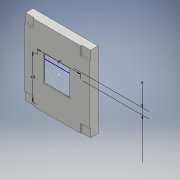
# Autodesk Inventor part: base
Saved by Autodesk Inventor 2018 (Build 220112000, 112)
## iProperties
Created: 2019-05-14
Part Number: base
Material: Generic
Document SubType Name: Modeling
Designer: jstklein
Density: 1 g/cm^3
Appearance: Default
Author: jstklein
Autodesk Inventor part; units mm, degrees
ref_plane "YZ Plane" through (0, 0, 0) normal (1, 0, 0) x (0, 1, 0)
ref_plane "XZ Plane" through (0, 0, 0) normal (0, 1, 0) x (-1, 0, 0)
ref_plane "XY Plane" through (0, 0, 0) normal (0, 0, 1) x (1, 0, 0)
sketch "Sketch1" plane through (0, 0, 0) normal (0, 1, 0) x (-1, 0, 0)
  line L0 (-30, 35) -> (30, 35)
  line L1 (30, 35) -> (30, -35)
  line L2 (30, -35) -> (-30, -35)
  line L3 (-30, -35) -> (-30, 35)
  line L4 (-30, 35) -> (30, -35) construction
  line L5 (30, 35) -> (-30, -35) construction
  point P0 (0, 0)
  dimension "d0" = 60
  dimension "d1" = 70
  constraints: 12 end point, 2 midpoint, 2 parallel, 1 horizontal, 1 perpendicular
  measures "d0" distance of L0.start L0.end
  measures "d1" distance of L0.end L1.end
extrude "Extrusion1" add sketch "Sketch1" along normal blind 8
sketch "Sketch2" plane through (0, 8, 0) normal (0, 1, 0) x (1, 0, 0)
  line L0 (27, -32) -> (27, 32)
  line L1 (27, 32) -> (-27, 32)
  line L2 (-27, 32) -> (-27, -32)
  line L3 (-27, -32) -> (27, -32)
  line L4 (27, -32) -> (-27, 32) construction
  line L5 (27, 32) -> (-27, -32) construction
  point P0 (0, 0)
  dimension "d4" = 64
  dimension "d5" = 54
  constraints: 12 end point, 2 midpoint, 2 parallel, 1 perpendicular, 1 vertical
  measures "d4" distance of L0.start L0.end
  measures "d5" distance of L1.end L0.end
extrude "Extrusion2" cut sketch "Sketch2" against normal blind 6
sketch "Sketch3" plane through (0, 2, 0) normal (0, 1, 0) x (1, 0, 0)
  line L0 (-12, -12) -> (12, -12)
  line L1 (12, -12) -> (12, 12)
  line L2 (12, 12) -> (-12, 12)
  line L3 (-12, 12) -> (-12, -12)
  line L4 (-12, -12) -> (12, 12) construction
  line L5 (12, -12) -> (-12, 12) construction
  line L6 (-13, -13) -> (13, -13)
  line L7 (13, -13) -> (13, 13)
  line L8 (13, 13) -> (-13, 13)
  line L9 (-13, 13) -> (-13, -13)
  line L10 (-13, -13) -> (13, 13) construction
  line L11 (13, -13) -> (-13, 13) construction
  circle A0 centre (-13, -13) radius 1.5
  circle A1 centre (-13, 13) radius 1.5
  circle A2 centre (13, 13) radius 1.5
  circle A3 centre (13, -13) radius 1.5
  point P0 (0, 0)
  dimension "d8" = 24
  dimension "d9" = 24
  dimension "d10" = 26
  dimension "d11" = 26
  dimension "d23" = 3
  dimension "d24" = 3
  dimension "d25" = 3
  dimension "d26" = 3
  constraints: 24 end point, 4 centre point, 4 coincident, 4 midpoint, 4 parallel, 2 horizontal, 2 perpendicular
  measures "d8" distance of L2.end L1.end
  measures "d9" distance of L1.end L0.end
  measures "d10" distance of L8.end L7.end
  measures "d11" distance of L7.end L6.end
  measures "d23" diameter of A0
  measures "d24" diameter of A1
  measures "d25" diameter of A2
  measures "d26" diameter of A3
extrude "Extrusion3" cut sketch "Sketch3" against normal blind 1.5
sketch "Sketch4" plane through (0, 0.5, 0) normal (0, 1, 0) x (1, 0, 0)
  line L0 (-12, -12) -> (12, -12)
  line L1 (12, -12) -> (12, 12)
  line L2 (12, 12) -> (-12, 12)
  line L3 (-12, 12) -> (-12, -12)
  line L4 (-12, -12) -> (12, 12) construction
  line L5 (12, -12) -> (-12, 12) construction
  point P0 (0, 0)
  dimension "d18" = 24
  dimension "d19" = 24
  constraints: 12 end point, 2 midpoint, 2 parallel, 1 horizontal, 1 perpendicular
  measures "d18" distance of L2.end L1.end
  measures "d19" distance of L1.end L0.end
extrude "Extrusion4" cut sketch "Sketch4" against normal up to next
sketch "Sketch5" plane through (0, 2, 0) normal (0, 1, 0) x (1, 0, 0)
  point P0 (0, 0)
sketch "Sketch6" plane through (0, 2, 0) normal (0, 1, 0) x (1, 0, 0)
  line L0 (20, 34) -> (-20, 34)
  line L1 (-20, 34) -> (-20, -6)
  line L2 (-20, -6) -> (20, -6)
  line L3 (20, -6) -> (20, 34)
  line L4 (20, 34) -> (-20, -6) construction
  line L5 (-20, 34) -> (20, -6) construction
  line L6 (12, -12) -> (-12, -12) projected
  point P0 (0, 0)
  point P1 (0, 14)
  dimension "d27" = 40
  dimension "d28" = 40
  dimension "d29" = 6
  constraints: 12 end point, 2 midpoint, 2 parallel, 1 horizontal, 1 perpendicular
  measures "d27" distance of L2.end L1.end
  measures "d28" distance of L1.end L0.end
  measures "d29" distance between parallel lines of L6 L2
sketch "Sketch7" plane through (0, 8, 0) normal (0, 1, 0) x (1, 0, 0)
  point P0 (0, 0)
sketch "Sketch8" plane through (0, 0, 0) normal (0, -1, 0) x (1, 0, 0)
  line L0 (-30, -35) -> (-30, 35) projected
  line L1 (-30, -35) -> (-22, -35)
  line L2 (-22, -35) -> (-22, -27)
  line L3 (-22, -27) -> (-30, -27)
  line L4 (-30, -27) -> (-30, -35)
  line L5 (-30, 35) -> (30, 35) projected
  line L6 (-30, 35) -> (-22, 35)
  line L7 (-22, 35) -> (-22, 27)
  line L8 (-22, 27) -> (-30, 27)
  line L9 (-30, 27) -> (-30, 35)
  line L10 (30, -35) -> (30, 35) projected
  line L11 (30, 35) -> (22, 35)
  line L12 (22, 35) -> (22, 27)
  line L13 (22, 27) -> (30, 27)
  line L14 (30, 27) -> (30, 35)
  line L15 (30, -35) -> (22, -35)
  line L16 (22, -35) -> (22, -27)
  line L17 (22, -27) -> (30, -27)
  line L18 (30, -27) -> (30, -35)
  point P0 (0, 0)
  dimension "d30" = 8
  dimension "d31" = 8
  dimension "d32" = 8
  dimension "d33" = 8
  dimension "d34" = 8
  dimension "d35" = 8
  dimension "d36" = 8
  dimension "d37" = 8
  constraints: 32 end point, 8 parallel, 4 horizontal, 4 perpendicular
  measures "d30" distance of L3.end L2.end
  measures "d31" distance of L2.end L1.end
  measures "d32" distance of L7.end L8.end
  measures "d33" distance of L6.end L7.end
  measures "d34" distance of L13.end L12.end
  measures "d35" distance of L12.end L11.end
  measures "d36" distance of L16.end L17.end
  measures "d37" distance of L15.end L16.end
extrude "Extrusion5" cut sketch "Sketch8" against normal blind 1
body "Solid1"
